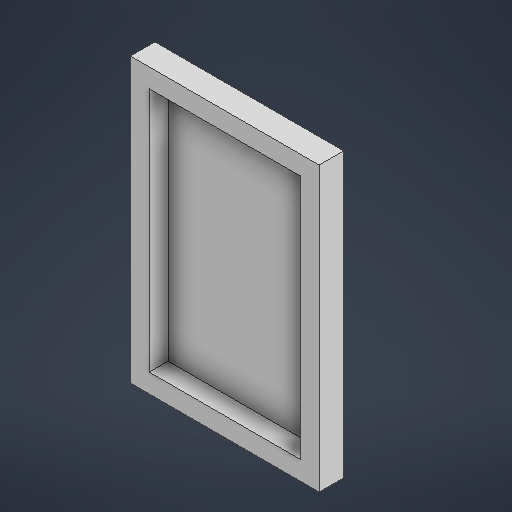
# Autodesk Inventor part: project2
Saved by Autodesk Inventor 2026 (Build 300175000, 175)
## iProperties
Created: 2026-09-09
Part Number: project2
Material: Типовые
Document SubType Name: Modeling
Designer: Roman
Density: 1 g/cm^3
Appearance: По умолчанию
Author: Roman
Autodesk Inventor part; units mm, degrees
ref_plane "YZ Plane" through (0, 0, 0) normal (1, 0, 0) x (0, 1, 0)
ref_plane "XZ Plane" through (0, 0, 0) normal (0, 1, 0) x (-1, 0, 0)
ref_plane "XY Plane" through (0, 0, 0) normal (0, 0, 1) x (1, 0, 0)
sketch "Эскиз1" plane through (0, 0, 0) normal (0, 0, 1) x (1, 0, 0)
  line L0 (50, -75) -> (-50, -75)
  line L1 (-50, -75) -> (-50, 75)
  line L2 (-50, 75) -> (50, 75)
  line L3 (50, 75) -> (50, -75)
  line L4 (50, -75) -> (-50, 75) construction
  line L5 (-50, -75) -> (50, 75) construction
  point P0 (0, 0)
  dimension "d0" = 100
  dimension "d1" = 150
  constraints: 12 end point, 2 midpoint, 2 parallel, 1 horizontal, 1 perpendicular
  measures "d0" distance between parallel lines of L3 L1
  measures "d1" distance between parallel lines of L0 L2
extrude "Выдавливание1" add sketch "Эскиз1" along normal blind 3
sketch "Эскиз2" plane through (0, 0, 3) normal (0, 0, 1) x (1, 0, 0)
  line L0 (-50, 75) -> (-50, -75) projected
  line L1 (50, -75) -> (-50, -75)
  line L2 (-50, -75) -> (-50, 75)
  line L3 (-50, 75) -> (50, 75)
  line L4 (50, 75) -> (50, -75)
  line L5 (50, -75) -> (-50, 75) construction
  line L6 (-50, -75) -> (50, 75) construction
  line L7 (-50.1414, 75) -> (-50.1414, -75)
  line L8 (40, 65) -> (-40, 65)
  line L9 (-40, 65) -> (-40, -65)
  line L10 (-40, -65) -> (40, -65)
  line L11 (40, -65) -> (40, 65)
  point P0 (0, 0)
  dimension "d4" = 10
  constraints: 22 end point, 5 parallel, 2 midpoint, 2 perpendicular, 1 horizontal, 3 other
  measures "d4" distance between parallel lines of L9 L0
extrude "Выдавливание2" add sketch "Эскиз2" along normal blind 10
sketch "Эскиз3" plane through (0, 0, 0) normal (1, 0, 0) x (0, 1, 0)
  line L0 (0, 0) -> (-75, -20.0962)
  line L1 (-75, 0) -> (75, 0) projected
  line L2 (-75, -20.0962) -> (-75, 0)
  line L3 (-75, 0) -> (0, 0)
  dimension "d7" = 15
  constraints: 6 end point, 2 perpendicular
  measures "d7" angle of L0 L1
extrude "Выдавливание3" add sketch "Эскиз3" along normal mid plane 20
